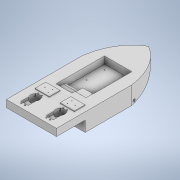
# Autodesk Inventor part: MainBody
Saved by Autodesk Inventor 2020.1 (Build 241239000, 239)
## iProperties
Created: 2021-12-15
Part Number: MainBody
Material: Generic
Document SubType Name: Modeling
Designer: OEM
Density: 1 g/cm^3
Appearance: Default
Author: OEM
Autodesk Inventor part; units mm, degrees
ref_plane "YZ Plane" through (0, 0, 0) normal (1, 0, 0) x (0, 1, 0)
ref_plane "XZ Plane" through (0, 0, 0) normal (0, 1, 0) x (-1, 0, 0)
ref_plane "XY Plane" through (0, 0, 0) normal (0, 0, 1) x (1, 0, 0)
sketch "Sketch1" plane through (0, 0, 0) normal (0, 1, 0) x (-1, 0, 0)
  line L0 (28.25, 20.4) -> (-28.25, 20.4) construction
  line L1 (-28.25, 20.4) -> (-28.25, -65.2) construction
  line L2 (-28.25, -65.2) -> (28.25, -65.2) construction
  line L3 (28.25, -65.2) -> (28.25, 20.4) construction
  line L4 (28.25, 20.4) -> (-28.25, -65.2) construction
  line L5 (-28.25, 20.4) -> (28.25, -65.2) construction
  line L6 (0, 600.8) -> (0, -638.2) construction
  spline S0 degree 2 poles (70, -42.8) (58.3679, -124.7541) (0, -160.2) knots 0 0 0 1 1 1
  line L7 (70, -42.8) -> (70, 157.2)
  line L8 (70, 157.2) -> (0, 157.2)
  spline S1 degree 2 poles (-70, -42.8) (-58.3679, -124.7541) (0, -160.2) knots 0 0 0 1 1 1
  line L9 (-70, -42.8) -> (-70, 157.2)
  line L10 (-70, 157.2) -> (0, 157.2)
  line L11 (70, 87.2) -> (-70, 87.2)
  line L12 (0, 87.2) -> (70, 157.2) construction
  line L13 (0, 157.2) -> (70, 87.2) construction
  circle A0 centre (35, 122.2) radius 12.5
  line L14 (0, 87.2) -> (-70, 157.2) construction
  line L15 (0, 157.2) -> (-70, 87.2) construction
  circle A1 centre (-35, 122.2) radius 12.5
  line L16 (-38.25, 30.4) -> (38.25, 30.4)
  line L17 (38.25, 30.4) -> (38.25, -75.2)
  line L18 (38.25, -75.2) -> (-38.25, -75.2)
  line L19 (-38.25, -75.2) -> (-38.25, 30.4)
  line L20 (-38.25, 30.4) -> (38.25, -75.2) construction
  line L21 (38.25, 30.4) -> (-38.25, -75.2) construction
  line L22 (-6.75, 20.4) -> (-6.75, -42.8) construction
  line L23 (-6.75, 20.4) -> (-6.75, 50.4) construction
  line L24 (-6.75, 50.4) -> (38.25, 50.4)
  line L25 (38.25, 50.4) -> (38.25, 30.4)
  line L26 (-6.75, 30.4) -> (-6.75, 50.4)
  circle A2 centre (24.75, -61.7) radius 1.125
  circle A3 centre (-24.75, -61.7) radius 1.125
  line L27 (-24.75, -61.7) -> (24.75, -61.7) construction
  line L28 (-24.75, -36.95) -> (24.75, -36.95) construction
  line L29 (-24.75, -36.95) -> (-24.75, -61.7) construction
  line L30 (24.75, -36.95) -> (24.75, -61.7) construction
  circle A4 centre (24.75, -12.2) radius 1.125
  circle A5 centre (-24.75, -12.2) radius 1.125
  line L31 (-24.75, -12.2) -> (24.75, -12.2) construction
  line L32 (-24.75, -36.95) -> (-24.75, -12.2) construction
  line L33 (24.75, -36.95) -> (24.75, -12.2) construction
  line L34 (-6.75, 30.4) -> (-38.25, 30.4)
  line L35 (-38.25, 30.4) -> (-38.25, 50.4) construction
  line L36 (-38.25, 50.4) -> (-6.75, 50.4) construction
  line L37 (-6.75, 50.4) -> (-6.75, 30.4)
  line L38 (-6.75, 30.4) -> (-37.23, 30.4)
  line L39 (-37.23, 30.4) -> (-37.23, 51.99)
  line L40 (-37.23, 51.99) -> (-6.75, 51.99)
  line L41 (-6.75, 51.99) -> (-6.75, 30.4)
  circle A6 centre (-34.69, 32.94) radius 0.75
  circle A7 centre (-20.085, 49.45) radius 0.75
  line L42 (-45, 112.2) -> (-45, 151.5)
  line L43 (-45, 151.5) -> (-25, 151.5)
  line L44 (-25, 112.2) -> (-25, 108.45) construction
  line L45 (-25, 108.45) -> (-45, 108.45) construction
  line L46 (-45, 108.45) -> (-45, 112.2) construction
  line L47 (-25, 112.2) -> (-25, 151.5)
  line L48 (-45, 112.2) -> (-25, 112.2)
  line L49 (-25, 151.5) -> (-45, 151.5)
  line L50 (-45, 151.5) -> (-45, 155.25) construction
  line L51 (-45, 155.25) -> (-25, 155.25) construction
  line L52 (-25, 155.25) -> (-25, 151.5) construction
  line L53 (70, 157.2) -> (-70, 157.2)
  line L54 (-70, 157.2) -> (-70, 167.2)
  line L55 (-70, 167.2) -> (70, 167.2)
  line L56 (70, 167.2) -> (70, 157.2)
  line L57 (-35, 108.45) -> (-35, 155.25) construction
  circle A8 centre (-30, 155.25) radius 2
  line L58 (-25, 131.85) -> (-45, 131.85) construction
  circle A9 centre (-40, 155.25) radius 2
  circle A10 centre (-30, 108.45) radius 2
  circle A11 centre (-40, 108.45) radius 2
  line L59 (45, 112.2) -> (45, 151.5)
  line L60 (45, 151.5) -> (25, 151.5)
  line L61 (25, 112.2) -> (25, 151.5)
  line L62 (45, 112.2) -> (25, 112.2)
  line L63 (45, 151.5) -> (45, 155.25) construction
  line L64 (45, 155.25) -> (25, 155.25) construction
  line L65 (25, 155.25) -> (25, 151.5) construction
  line L66 (35, 108.45) -> (35, 155.25) construction
  circle A12 centre (30, 155.25) radius 2
  circle A13 centre (40, 155.25) radius 2
  circle A14 centre (30, 108.45) radius 2
  circle A15 centre (40, 108.45) radius 2
  line L67 (45, 108.45) -> (25, 108.45) construction
  line L68 (45, 108.45) -> (45, 112.2) construction
  line L69 (25, 108.45) -> (25, 112.2) construction
  line L70 (-72.4135, -25.7958) -> (-67.5865, -59.8042) construction
  arc A16 (-71.5687, -29.1646) -> (-67.7125, -56.3334) centre (186.925, -6.3334) ccw construction
  line L71 (-15, 102.2) -> (-55, 102.2)
  line L72 (-55, 102.2) -> (-55, 72.2)
  line L73 (-55, 72.2) -> (-15, 72.2)
  line L74 (-15, 72.2) -> (-15, 102.2)
  line L75 (-15, 102.2) -> (-55, 72.2) construction
  line L76 (-55, 102.2) -> (-15, 72.2) construction
  line L77 (15, 102.2) -> (55, 102.2)
  line L78 (55, 102.2) -> (55, 72.2)
  line L79 (55, 72.2) -> (15, 72.2)
  line L80 (15, 72.2) -> (15, 102.2)
  circle A17 centre (26.8629, 81.1136) radius 0.75
  circle A18 centre (42.4108, 87.2) radius 0.75
  circle A19 centre (26.8629, 93.2864) radius 0.75
  circle A20 centre (-26.8629, 81.1136) radius 0.75
  circle A21 centre (-42.4108, 87.2) radius 0.75
  circle A22 centre (-26.8629, 93.2864) radius 0.75
  point P0 (0, -22.4)
  point P1 (44.8, -116.1993)
  point P2 (-44.8, -116.1993)
  point P3 (25, 129.7)
  point P4 (45, 129.7)
  point P5 (27.5, 112.2)
  point P6 (25, 114.7)
  point P7 (42.5, 112.2)
  point P8 (45, 114.7)
  point P9 (-42.5, 112.2)
  point P10 (-45, 114.7)
  point P11 (-27.5, 112.2)
  point P12 (-25, 114.7)
  point P13 (-25, 129.7)
  point P14 (-45, 129.7)
  point P15 (-35, 87.2)
  dimension "d1" = 85.6
  dimension "d5" = 25
  dimension "d6" = 10
  dimension "d7" = 10
  dimension "d17" = 89.6
  dimension "d29" = 56.5
  dimension "d30" = 70
  dimension "d31" = 35
  dimension "d32" = 20
  dimension "d37" = 3.5
  dimension "d38" = 3.5
  dimension "d40" = 2.25
  dimension "d43" = 24.75
  dimension "d48" = 21.59
  dimension "d49" = 30.48
  dimension "d50" = 1.5
  dimension "d51" = 2.54
  dimension "d52" = 2.54
  dimension "d53" = 2.54
  dimension "d54" = 14.605
  dimension "d63" = 3.75
  dimension "d64" = 10
  dimension "d66" = 3.75
  dimension "d68" = 39.3
  dimension "d69" = 90
  dimension "d70" = 20
  dimension "d71" = 10
  dimension "d72" = 10
  dimension "d74" = 5
  dimension "d75" = 4
  dimension "d76" = 19.65
  dimension "d82" = 247.4
  dimension "d83" = 130
  dimension "d86" = 70
  dimension "d87" = 10
  dimension "d88" = 85
  dimension "d90" = 10
  dimension "d92" = 24.75
  dimension "d95" = 140
  dimension "d96" = 73.3993
  dimension "d97" = 38.25
  dimension "d98" = 10
  dimension "d99" = 35.921
  dimension "d100" = 33.427
  dimension "d101" = 90
  dimension "d102" = 90
  dimension "d105" = 1.5
  dimension "d106" = 6.0864
  dimension "d107" = 11.8628
  dimension "d108" = 1.5
  dimension "d109" = 15.548
  dimension "d115" = 1.5
  constraints: 162 end point, 31 symmetric about line, 23 centre point, 17 parallel, 14 midpoint, 11 perpendicular, 10 point on line, 8 horizontal, 7 vertical, 1 collinear, 1 point on circle, 24 other
  measures "d1" distance of L1.end L0.end
  measures "d5" diameter of A0
  measures "d6" distance between parallel lines of L16 L0
  measures "d7" distance between parallel lines of L17 L3
  measures "d17" diameter of point (44.8, -116.199) L6
  measures "d29" distance between parallel lines of L1 L3
  measures "d30" distance between parallel lines of L6 L7
  measures "d31" distance between parallel lines of L22 L3
  measures "d32" distance between parallel lines of L16 L24
  measures "d37" distance from line of L2 A2.centre
  measures "d38" distance from line of L3 A2.centre
  measures "d40" diameter of A2
  measures "d43" distance between parallel lines of L27 L28
  measures "d48" distance of L38.end L39.end
  measures "d49" distance of L39.end L40.end
  measures "d50" diameter of A6
  measures "d51" distance from line of L39 A6.centre
  measures "d52" distance from line of L16 A6.centre
  measures "d53" distance from line of L40 A7.centre
  measures "d54" horizontal distance of A6.centre A7.centre
  measures "d63" distance of L45.end L42.start
  measures "d64" horizontal distance of A1.centre L42.start
  measures "d66" distance of L42.end L50.end
  measures "d68" distance of L44.start L43.end
  measures "d69" angle of L42 L49
  measures "d70" distance of L44.end L45.end
  measures "d71" distance from line of L42 A1.centre
  measures "d72" distance from line of L47 A1.centre
  measures "d74" distance from line of L57 A8.centre
  measures "d75" diameter of A8
  measures "d76" distance of L44.start L58.start
  measures "d82" distance from line of L11 point (0, -160.2)
  measures "d83" distance of L11.end L9.start
  measures "d86" distance of L11.end L9.end
  measures "d87" distance of L53.end L54.end
  measures "d88" distance from line of point (0, -160.2) L18
  measures "d90" distance between parallel lines of L19 L1
  measures "d92" distance from line of L33 point (0, -22.4)
  measures "d95" distance of L7.start L9.start
  measures "d96" vertical distance of L9.start point (-44.8, -116.199)
  measures "d97" distance between parallel lines of L17 L6
  measures "d98" distance between parallel lines of L18 L2
  measures "d99" angle of L17 L20
  measures "d100" angle of L3 L5
  measures "d101" angle of L27 L29
  measures "d102" angle of L27 L30
  measures "d105" diameter of A17
  measures "d106" distance from line of L11 A17.centre
  measures "d107" distance from line of L80 A17.centre
  measures "d108" diameter of A18
  measures "d109" horizontal distance of A17.centre A18.centre
  measures "d115" diameter of A7
extrude "Extrusion1" add sketch "Sketch1" against normal blind 50 contours S0 S1 L9 L11 L72 L73 L74 L80 L79 L78 L7 | L78 L79 L80 L11 A18 | A18 L11 | L11 A21 L74 L73 L72 | L11 A21 | L16 L17 L18 L19 | L39 L40 L41 L26 L16 | L26 L24 L25 L16 | A2 | A3 | A4 | A5 | A6 | A7 | A17 | A20 picked at (42.4409, 86.9518) picked at (-42.3807, 86.9518)
extrude "Extrusion2" add sketch "Sketch1" against normal blind 20 contours L11 L78 L77 L80 L74 L71 L72 L9 L10 A9 A8 L8 A12 A13 L7 | L8 A13 A12 L10 A8 A9 L54 L55 L56 | L11 A18 L80 L77 L78 | A13 L8 | L8 A13 | L11 A18 | L72 L71 L74 L11 A21 | A9 L10 | L10 A9 | A21 L11 | A12 L8 | L8 A12 | A8 L10 | L10 A8 | A0 L61 L60 L59 | L59 L62 A0 | A0 L62 L61 | A1 L42 L43 L47 | L47 L48 A1 | A1 L48 L42 | A10 | A11 | A14 | A15 | A19 | A22 picked at (42.4409, 87.4482) picked at (-42.3807, 87.4482)
extrude "Extrusion3" cut sketch "Sketch1" against normal blind 20 contours L16 L17 L18 L19 | A2 | A3 | A4 | A5
sketch "Sketch2" plane through (70, -50, -42.8) normal (1, 0, 0) x (0, 0, -1)
  line L0 (0, 50) -> (0, 0) projected
  line L1 (0, 0) -> (89, 11) construction
  line L2 (117.4, 50) -> (117.4, 0) projected
  line L3 (89, 11) -> (117.4, 50) construction
  spline S0 degree 2 poles (0, 0) (89, 11) (117.4, 50) knots 1 1 1 2 2 2
  line L4 (-130, 0) -> (0, 0) projected
  line L5 (0, 0) -> (117.4, 0)
  point P0 (-42.8, 50)
  constraints: 2 end point, 1 collinear, 3 other
extrude "Extrusion4" cut sketch "Sketch2" against normal blind 200
sketch "Sketch3" plane through (70, -50, 87.2) normal (1, 0, 0) x (0, 0, -1)
  circle A0 centre (138, 8) radius 3.6056
  line L0 (130, 50) -> (130, 0) projected
  line L1 (0, 0) -> (130, 0) construction
  line L2 (0, 0) -> (300, 0) construction
  point P0 (87.2, 50)
  dimension "d18" = 8
  dimension "d19" = 8
  constraints: 2 end point, 1 centre point, 1 collinear
  measures "d18" distance from line of L0 A0.centre
  measures "d19" distance from line of L2 A0.centre
extrude "Extrusion5" cut sketch "Sketch3" against normal blind 200
extrude "Extrusion6" cut sketch "Sketch1" against normal blind 10 contours L26 L24 L25 L16
fillet "Fillet1" radius 10 1 edges at (-15.75, -10, 30.4)
fillet "Fillet2" radius 10 1 edges at (-15.75, 0, 50.4) inverted yes
extrude "RPi_mounting_holes" cut sketch "Sketch1" against normal blind 26 contours A2 | A3 | A4 | A5
extrude "Extrusion8" cut sketch "Sketch1" against normal blind 2 contours L39 L40 L41 L26 L16
extrude "Maestro_mounting_holes" cut sketch "Sketch1" against normal blind 6 contours A6 | A7
extrude "Extrusion10" cut sketch "Sketch1" against normal blind 7 contours A0 L61 L60 L59 | L59 L62 A0 | A0 L62 L61 | A1 L42 L43 L47 | L47 L48 A1 | A1 L48 L42
extrude "Servo_mounting_holes" cut sketch "Sketch1" against normal blind 10 contours A13 L8 | L8 A13 | A9 L10 | L10 A9 | A12 L8 | L8 A12 | A8 L10 | L10 A8 | A10 | A11 | A14 | A15
extrude "Extrusion12" add sketch "Sketch1" along normal blind 2 contours L78 L79 L80 L11 A18 | L11 A18 L80 L77 L78 | A18 L11 | L11 A18 | L72 L71 L74 L11 A21 | L11 A21 L74 L73 L72 | A21 L11 | L11 A21 | A17 | A19 | A20 | A22
extrude "Motor_Controller_mounting_holes" cut sketch "Sketch1" along normal blind 2 and the other way blind 4 contours A18 L11 | L11 A18 | A21 L11 | L11 A21 | A17 | A19 | A20 | A22
equation "\"d43\" = 0.5 * d41"
equation "\"d71\" = 0.5 * d70"
equation "\"d72\" = 0.5 * d70"
equation "\"d76\" = 0.5 * d68"
equation "\"d41\" = 49.5"
body "Solid1"
